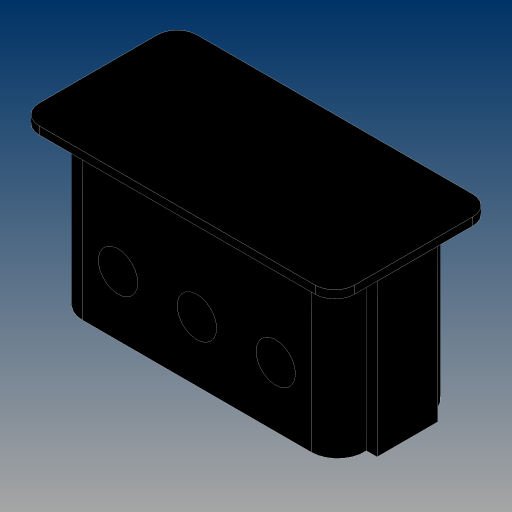
# Autodesk Inventor part: ELEV_015_CRSHBLCK1
Saved by Autodesk Inventor 2024.3 (Build 283343000, 343)
## iProperties
Created: 2024-11-27
Part Number: ELEV_015_CRSHBLCK1
Material: ABS Plastic
Document SubType Name: Modeling
Designer: Kenji
Density: 1.06 g/cm^3
Appearance: Anodized - Black
Author: Kenji
Autodesk Inventor part; units mm, degrees
ref_plane "YZ Plane" through (0, 0, 0) normal (1, 0, 0) x (0, 1, 0)
ref_plane "XZ Plane" through (0, 0, 0) normal (0, 1, 0) x (-1, 0, 0)
ref_plane "XY Plane" through (0, 0, 0) normal (0, 0, 1) x (1, 0, 0)
sketch "Sketch1" plane through (0, 0, 0) normal (0, 1, 0) x (-1, 0, 0)
  line L0 (0, -4.6482) -> (0, -14.4272)
  line L1 (5.9563, -19.05) -> (42.8117, -19.05)
  line L2 (48.768, -14.4272) -> (48.768, -4.6482)
  line L3 (42.8117, 0) -> (5.9563, 0)
  line L4 (0, -14.4272) -> (1.7272, -14.4272)
  line L5 (48.768, -4.6482) -> (47.0408, -4.6482)
  line L6 (48.768, -14.4272) -> (47.0408, -14.4272)
  line L7 (0, -4.6482) -> (1.7272, -4.6482)
  line L8 (24.384, 0) -> (24.384, -19.05) construction
  arc A0 (5.9563, 0) -> (1.7272, -4.6482) centre (5.9563, -4.248) ccw
  arc A1 (1.7272, -14.4272) -> (5.9563, -19.05) centre (5.9586, -14.802) ccw
  arc A2 (47.0408, -4.6482) -> (42.8117, 0) centre (42.8117, -4.248) ccw
  arc A3 (42.8117, -19.05) -> (47.0408, -14.4272) centre (42.8094, -14.802) ccw
  point P0 (0, 0)
  dimension "d1" = 19.05
  dimension "d2" = 48.768
  dimension "d3" = 36.8554
  dimension "d4" = 1.7272
  dimension "d6" = 9.779
  dimension "d8" = 24.384
  dimension "d9" = 4.6482
  constraints: 18 end point, 8 point on circle, 5 equal length, 5 horizontal, 4 centre point, 3 equal radius, 2 horizontal alignment, 2 midpoint, 2 point on line, 2 tangent, 2 vertical alignment, 1 perpendicular, 1 vertical
  measures "d1" distance between parallel lines of L1 L3
  measures "d2" distance between parallel lines of L0 L2
  measures "d3" distance of L3.start L3.end
  measures "d4" distance of L0.start L7.end
  measures "d6" distance of L2.start L2.end
  measures "d8" distance between parallel lines of L8 L2
  measures "d9" distance between parallel lines of L5 L3
extrude "Extrusion1" add sketch "Sketch1" along normal blind 25.527
sketch "Sketch2" plane through (0, 25.527, 0) normal (0, 1, 0) x (1, 0, 0)
  line L0 (-46.609, -3.175) -> (-2.159, -3.175)
  line L1 (1.016, 0) -> (1.016, 19.05)
  line L2 (-2.159, 22.225) -> (-46.609, 22.225)
  line L3 (-49.784, 19.05) -> (-49.784, 0)
  line L4 (-5.9563, 19.05) -> (-42.8117, 19.05) projected
  line L5 (-48.768, 14.4272) -> (-48.768, 4.6482) projected
  line L6 (-42.8117, 0) -> (-5.9563, 0) projected
  line L7 (0, 4.6482) -> (0, 14.4272) projected
  arc A0 (-49.784, 0) -> (-46.609, -3.175) centre (-46.609, 0) ccw
  arc A1 (-46.609, 22.225) -> (-49.784, 19.05) centre (-46.609, 19.05) ccw
  arc A2 (1.016, 19.05) -> (-2.159, 22.225) centre (-2.159, 19.05) ccw
  arc A3 (-2.159, -3.175) -> (1.016, 0) centre (-2.159, 0) ccw
  point P0 (0, 0)
  point P1 (-49.784, -3.175)
  point P2 (1.016, 22.225)
  point P3 (-49.784, 22.225)
  dimension "d13" = 3.175
  dimension "d16" = 1.016
  dimension "d17" = 25.4
  dimension "d18" = 50.8
  dimension "d19" = 3.175
  constraints: 8 end point, 8 point on circle, 8 tangent, 6 point on line, 4 centre point, 3 equal radius, 2 parallel, 1 horizontal, 1 perpendicular
  measures "d13" distance between parallel lines of L4 L2
  measures "d16" distance between parallel lines of L1 L7
  measures "d17" distance of point (-49.784, 22.225) point (-49.784, -3.175)
  measures "d18" distance of point (1.016, 22.225) point (-49.784, 22.225)
  measures "d19" radius of A0
extrude "Extrusion2" add sketch "Sketch2" along normal blind 1.27
sketch "Sketch3" plane through (-42.8117, 0, 0) normal (0, 0, 1) x (1, 0, 0)
  circle A0 centre (5.7277, 9.652) radius 3.175
  circle A1 centre (18.4277, 9.652) radius 3.175
  circle A2 centre (31.1277, 9.652) radius 3.175
  line L0 (-5.9563, 0) -> (-5.9563, 25.527) projected
  line L1 (0, 25.527) -> (36.8554, 25.527) projected
  point P0 (42.8117, 0)
  point P1 (43.8277, 25.527)
  point P2 (-6.9723, 25.527)
  dimension "d22" = 12.7
  dimension "d23" = 12.7
  dimension "d25" = 15.875
  dimension "d26" = 6.35
  dimension "d29" = 12.7
  constraints: 3 centre point, 2 equal radius, 2 horizontal alignment
  measures "d22" distance of A1.centre A0.centre
  measures "d23" distance of A2.centre A1.centre
  measures "d25" distance from line of L1 A0.centre
  measures "d26" diameter of A0
  measures "d29" horizontal distance of A2.centre point (43.828, 25.527)
extrude "Extrusion3" cut sketch "Sketch3" against normal through all
equation "\"d8\" = 0.5 * d2"
body "Solid1"
